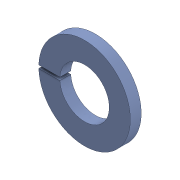
# Autodesk Inventor part: Arandela Grower M4 - DMI
Saved by Autodesk Inventor 2020.3 (Build 243373000, 373)
## iProperties
Created: 2020-05-19
Part Number: Arandela Grower M4 - DMI
Material: Generic
Document SubType Name: Modeling
Designer: Dante
Density: 1 g/cm^3
Appearance: Rubber - Blue
Author: Dante
Autodesk Inventor part; units mm, degrees
ref_plane "YZ Plane" through (0, 0, 0) normal (1, 0, 0) x (0, 1, 0)
ref_plane "XZ Plane" through (0, 0, 0) normal (0, 1, 0) x (-1, 0, 0)
ref_plane "XY Plane" through (0, 0, 0) normal (0, 0, 1) x (1, 0, 0)
sketch "Sketch1" plane through (0, 0, 0) normal (0, 0, 1) x (1, 0, 0)
  circle A0 centre (0, 0) radius 2.05
  circle A1 centre (0, 0) radius 3.8
  line L0 (-4, 0.125) -> (-4, -0.125)
  line L1 (-4, -0.125) -> (0, -0.125)
  line L2 (0, -0.125) -> (0, 2.952)
  line L3 (-4, 0.125) -> (1.123, 0.125)
  point P0 (-3.7979, 0.125)
  point P1 (-2.0462, 0.125)
  point P2 (-2.0462, -0.125)
  point P3 (-3.7979, -0.125)
  dimension "d0" = 4.1
  dimension "d1" = 7.6
  dimension "d2" = 0.125
  dimension "d4" = 0.125
  constraints: 8 end point, 2 centre point, 2 coincident, 1 horizontal, 1 perpendicular
  measures "d0" diameter of A0
  measures "d1" diameter of A1
  measures "d2" distance from line of L3 point (0, 0)
  measures "d4" distance from line of point (0, 0) L1
extrude "Extrusion1" add sketch "Sketch1" along normal blind 0.9 contours A0 L3 A1 L1 picked at (3.1615, -0.4604)
body "Solid1"
